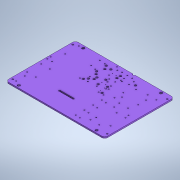
# Autodesk Inventor part: Internal Rear Plate
Saved by Autodesk Inventor 2021 (Build 250183000, 183)
## iProperties
Created: 2020-07-02
Part Number: Internal Rear Plate
Material: Generic
Document SubType Name: Modeling
Designer: jgray
Density: 1 g/cm^3
Appearance: Default
Author: jgray
Autodesk Inventor part; units mm, degrees
ref_plane "YZ Plane" through (0, 0, 0) normal (1, 0, 0) x (0, 1, 0)
ref_plane "XZ Plane" through (0, 0, 0) normal (0, 1, 0) x (-1, 0, 0)
ref_plane "XY Plane" through (0, 0, 0) normal (0, 0, 1) x (1, 0, 0)
sketch "Sketch1" plane through (0, 0, 0) normal (0, 1, 0) x (-1, 0, 0)
  line L0 (165, -123) -> (-165, -123)
  line L1 (-175, -113) -> (-175, 113)
  line L2 (-165, 123) -> (165, 123)
  line L3 (175, 113) -> (175, -113)
  line L4 (175, -123) -> (-175, 123) construction
  line L5 (-175, -123) -> (175, 123) construction
  arc A0 (165, -123) -> (175, -113) centre (165, -113) ccw
  arc A1 (175, 113) -> (165, 123) centre (165, 113) ccw
  arc A2 (-165, 123) -> (-175, 113) centre (-165, 113) ccw
  arc A3 (-175, -113) -> (-165, -123) centre (-165, -113) ccw
  line L6 (-137.85, 113.9) -> (137.85, 113.9) construction
  line L7 (137.85, 113.9) -> (137.85, -113.9) construction
  line L8 (137.85, -113.9) -> (-137.85, -113.9) construction
  line L9 (-137.85, -113.9) -> (-137.85, 113.9) construction
  line L10 (-137.85, 113.9) -> (137.85, -113.9) construction
  line L11 (137.85, 113.9) -> (-137.85, -113.9) construction
  line L12 (137.85, -114.5) -> (137.85, -113.3) construction
  line L13 (142.05, -114.5) -> (142.05, -113.3)
  line L14 (133.65, -113.3) -> (133.65, -114.5)
  arc A4 (133.65, -114.5) -> (142.05, -114.5) centre (137.85, -114.5) ccw
  arc A5 (142.05, -113.3) -> (133.65, -113.3) centre (137.85, -113.3) ccw
  line L15 (137.85, 113.75) -> (137.85, 114.95) construction
  line L16 (142.05, 113.75) -> (142.05, 114.95)
  line L17 (133.65, 114.95) -> (133.65, 113.75)
  arc A6 (133.65, 113.75) -> (142.05, 113.75) centre (137.85, 113.75) ccw
  arc A7 (142.05, 114.95) -> (133.65, 114.95) centre (137.85, 114.95) ccw
  line L18 (-137.85, 113.75) -> (-137.85, 114.95) construction
  line L19 (-133.65, 113.75) -> (-133.65, 114.95)
  line L20 (-142.05, 114.95) -> (-142.05, 113.75)
  arc A8 (-142.05, 113.75) -> (-133.65, 113.75) centre (-137.85, 113.75) ccw
  arc A9 (-133.65, 114.95) -> (-142.05, 114.95) centre (-137.85, 114.95) ccw
  line L21 (-137.85, -114.95) -> (-137.85, -113.75) construction
  line L22 (-133.65, -114.95) -> (-133.65, -113.75)
  line L23 (-142.05, -113.75) -> (-142.05, -114.95)
  arc A10 (-142.05, -114.95) -> (-133.65, -114.95) centre (-137.85, -114.95) ccw
  arc A11 (-133.65, -113.75) -> (-142.05, -113.75) centre (-137.85, -113.75) ccw
  point P0 (0, 0)
  point P1 (0, 0)
  point P2 (137.85, 114.35)
  point P3 (-137.85, 114.35)
  point P4 (-137.85, -114.35)
  dimension "d31" = 350
  dimension "d32" = 246
  dimension "d33" = 10
  dimension "d34" = 275.7
  dimension "d35" = 227.8
  dimension "d396" = 8.4
  dimension "d397" = 0.6
  dimension "d398" = 8.4
  dimension "d399" = 0.6
  dimension "d400" = 8.4
  dimension "d401" = 0.6
  dimension "d402" = 8.4
  dimension "d403" = 0.6
  dimension "d404" = 9.1
  dimension "d405" = 9.1
  constraints: 56 end point, 24 point on circle, 24 tangent, 12 centre point, 9 point on line, 8 parallel, 4 midpoint, 3 equal radius, 2 horizontal, 2 perpendicular
  measures "d31" distance of L4.start L5.start
  measures "d32" distance between parallel lines of L0 L2
  measures "d33" radius of A0
  measures "d34" distance of L7.end L8.end
  measures "d35" distance of L6.end L7.end
  measures "d396" diameter of A5
  measures "d397" distance of L12.end L7.end
  measures "d398" diameter of A7
  measures "d399" distance of L15.end point (137.85, 114.35)
  measures "d400" diameter of A9
  measures "d401" distance of L18.end point (-137.85, 114.35)
  measures "d402" diameter of A11
  measures "d403" distance of L21.end point (-137.85, -114.35)
  measures "d404" distance between parallel lines of L2 L6
  measures "d405" distance between parallel lines of L0 L8
extrude "Extrusion1" add sketch "Sketch1" along normal blind 5
sketch "Sketch2" plane through (0, 5, 0) normal (0, 1, 0) x (1, 0, 0)
  line L0 (-165, -123) -> (165, -123) projected
  arc A0 (165, -123) -> (175, -113) centre (165, -113) ccw projected
  line L1 (175, -113) -> (175, 113) projected
  arc A1 (175, 113) -> (165, 123) centre (165, 113) ccw projected
  line L2 (165, 123) -> (-165, 123) projected
  arc A2 (-165, 123) -> (-175, 113) centre (-165, 113) ccw projected
  line L3 (-175, 113) -> (-175, -113) projected
  arc A3 (-175, -113) -> (-165, -123) centre (-165, -113) ccw projected
  line L4 (167.5, -106.5) -> (-167.5, -106.5)
  line L5 (-167.5, -106.5) -> (-167.5, 106.5)
  line L6 (-167.5, 106.5) -> (167.5, 106.5)
  line L7 (167.5, 106.5) -> (167.5, -106.5)
  line L8 (167.5, -106.5) -> (-167.5, 106.5) construction
  line L9 (-167.5, -106.5) -> (167.5, 106.5) construction
  point P0 (0, 0)
  dimension "d40" = 335
  dimension "d41" = 213
  constraints: 12 end point, 4 coincident, 2 midpoint, 2 parallel, 1 horizontal, 1 perpendicular
  measures "d40" distance of L5.end L6.end
  measures "d41" distance of L4.end L5.end
hole "Hole1" at (-167.5, 5, -106.5) at (167.5, 5, -106.5) at (167.5, 5, 106.5) at (-167.5, 5, 106.5) direction (0, -1, 0) diameter 5.6 end through all
sketch "Sketch5" plane through (0, 5, 0) normal (0, 1, 0) x (1, 0, 0)
  line L0 (150.75, 85) -> (119.75, 85) construction
  line L1 (119.75, -25) -> (150.75, -25) construction
  line L2 (199.9056, 0) -> (-194.4013, 0) construction
  line L3 (175, -113) -> (175, 113) projected
  point P0 (0, 0)
  point P1 (158, 0)
  dimension "d72" = 31
  dimension "d106" = 85
  dimension "d107" = 25
  dimension "d108" = 31
  dimension "d109" = 24.25
  dimension "d110" = 24.25
  constraints: 6 end point, 4 coincident, 2 horizontal, 2 point on line
  measures "d72" distance of L1.end L1.start
  measures "d106" distance from line of point (150.75, 85) L2
  measures "d107" distance between parallel lines of L2 L1
  measures "d108" distance of L0.start L0.end
  measures "d109" distance from line of L3 point (150.75, 85)
  measures "d110" distance from line of L3 point (150.75, -25)
hole "Hole3" at (150.75, 5, -85) at (119.75, 5, -85) at (150.75, 5, 25) at (119.75, 5, 25) direction (0, -1, 0) diameter 3.8 end through all
sketch "Sketch6" plane through (0, 5, 0) normal (0, 1, 0) x (1, 0, 0)
  line L0 (195.402, -93) -> (-63.7996, -93) construction
  line L1 (204.9094, 9) -> (-63.7996, 9) construction
  line L2 (-165, -123) -> (165, -123) construction
  line L3 (165, 123) -> (-165, 123) construction
  line L4 (175, -113) -> (175, 113) construction
  point P0 (0, 0)
  point P1 (195.402, -93)
  point P2 (-63.7996, -93)
  point P3 (204.9094, 9)
  point P4 (-63.7996, 9)
  point P5 (94.75, 9)
  point P6 (94.75, -93)
  point P7 (125.75, 9)
  point P8 (125.75, -93)
  dimension "d82" = 30
  dimension "d83" = 114
  dimension "d84" = 80.25
  dimension "d85" = 80.25
  dimension "d86" = 31
  dimension "d87" = 31
  dimension "d133" = 102
  constraints: 10 other
  measures "d84" distance from line of L4 point (94.75, 9)
  measures "d85" distance from line of point (94.75, -93) L4
  measures "d86" distance of point (94.75, 9) point (125.75, 9)
  measures "d87" distance of point (94.75, -93) point (125.75, -93)
  measures "d133" distance of point (125.75, -93) point (125.75, 9)
hole "Hole4" at (94.75, 5, -9) at (94.75, 5, 93) at (125.75, 5, -9) at (125.75, 5, 93) direction (0, -1, 0) diameter 3.8 end through all
sketch "Sketch7" plane through (0, 5, 0) normal (0, 1, 0) x (1, 0, 0)
  line L0 (-55.6475, -59) -> (-200.9918, -59) construction
  line L1 (-55.6475, -9) -> (-204.5492, -9) construction
  line L2 (-133.25, -141.7869) -> (-133.25, 81.8197) construction
  line L3 (-164.25, -146.3607) -> (-164.25, 53.8689) construction
  line L4 (-175, 113) -> (-175, -113) construction
  line L5 (-165, -123) -> (165, -123) construction
  point P0 (0, 0)
  point P1 (-164.25, -9)
  point P2 (-133.25, -9)
  point P3 (-133.25, -59)
  point P4 (-164.25, -59)
  dimension "d95" = 31
  dimension "d96" = 41.75
  dimension "d97" = 64
  dimension "d98" = 50
  constraints: 8 end point, 8 point on line, 2 horizontal, 2 vertical
  measures "d95" distance between parallel lines of L3 L2
  measures "d96" distance between parallel lines of L4 L2
  measures "d97" distance between parallel lines of L5 L0
  measures "d98" distance between parallel lines of L0 L1
hole "Hole5" at (-164.25, 5, 9) at (-133.25, 5, 9) at (-133.25, 5, 59) at (-164.25, 5, 59) direction (0, -1, 0) diameter 3.8 end through all
sketch "Sketch8" plane through (0, 5, 0) normal (0, 1, 0) x (1, 0, 0)
  line L0 (-156.25, -168.1311) -> (-156.25, 234.4364) construction
  line L1 (-175, 113) -> (-175, -113) construction
  line L2 (-165, -123) -> (165, -123) construction
  point P0 (0, 0)
  point P1 (-156.25, -106)
  point P2 (-156.25, -75)
  dimension "d111" = 18.75
  dimension "d112" = 17
  dimension "d113" = 31
  constraints: 2 end point, 2 point on line, 1 vertical
  measures "d111" distance between parallel lines of L1 L0
  measures "d112" distance from line of point (-156.25, -106) L2
  measures "d113" distance of point (-156.25, -75) point (-156.25, -106)
hole "Hole6" at (-156.25, 5, 106) at (-156.25, 5, 75) direction (0, -1, 0) diameter 3.8 end through all
sketch "Sketch9" plane through (0, 5, 0) normal (0, 1, 0) x (1, 0, 0)
  line L0 (69.75, 186.0812) -> (69.75, -151.0812) construction
  circle A0 centre (-156.25, -106) radius 1.9 construction
  circle A1 centre (-156.25, -75) radius 1.9 construction
  circle A2 centre (-133.25, -59) radius 1.9 construction
  circle A3 centre (-164.25, -9) radius 1.9 construction
  circle A4 centre (-133.25, -9) radius 1.9 construction
  circle A5 centre (-164.25, -59) radius 1.9 construction
  circle A6 centre (125.75, 9) radius 1.9 construction
  circle A7 centre (94.75, 9) radius 1.9 construction
  circle A8 centre (94.75, -93) radius 1.9 construction
  circle A9 centre (125.75, -93) radius 1.9 construction
  circle A10 centre (150.75, -25) radius 1.9 construction
  circle A11 centre (150.75, 85) radius 1.9 construction
  circle A12 centre (119.75, 85) radius 1.9 construction
  circle A13 centre (119.75, -25) radius 1.9 construction
  circle A14 centre (167.5, -106.5) radius 2.8 construction
  circle A15 centre (-167.5, 106.5) radius 2.8 construction
  circle A16 centre (167.5, 106.5) radius 2.8 construction
  circle A17 centre (-167.5, -106.5) radius 2.8 construction
  line L1 (-165, -123) -> (165, -123) construction
  arc A18 (165, -123) -> (175, -113) centre (165, -113) ccw construction
  line L2 (175, -113) -> (175, 113) construction
  arc A19 (175, 113) -> (165, 123) centre (165, 113) ccw construction
  line L3 (165, 123) -> (-165, 123) construction
  arc A20 (-165, 123) -> (-175, 113) centre (-165, 113) ccw construction
  line L4 (-175, 113) -> (-175, -113) construction
  arc A21 (-175, -113) -> (-165, -123) centre (-165, -113) ccw construction
  point P0 (0, 0)
  point P1 (69.75, -106)
  point P2 (69.75, -75)
  point P3 (69.75, 17.5)
  point P4 (69.75, 48.5)
  dimension "d121" = 226
  dimension "d122" = 17
  dimension "d123" = 31
  dimension "d131" = 123.5
  dimension "d132" = 31
  constraints: 3 point on line, 2 end point, 1 midpoint, 1 vertical
  measures "d121" distance from line of A0.centre L0
  measures "d122" distance from line of point (69.75, -106) L1
  measures "d123" distance of point (69.75, -75) point (69.75, -106)
  measures "d131" distance of point (69.75, 17.5) point (69.75, -106)
  measures "d132" distance of point (69.75, 48.5) point (69.75, 17.5)
hole "Hole7" at (69.75, 5, 106) at (69.75, 5, 75) at (69.75, 5, -48.5) at (69.75, 5, -17.5) direction (0, -1, 0) diameter 3.8 end through all
sketch "Sketch10" plane through (0, 5, 0) normal (0, 1, 0) x (1, 0, 0)
  line L0 (-152.5, 188.1856) -> (-152.5, -152.5856) construction
  line L1 (-175, 113) -> (-175, -113) construction
  line L2 (-244.4549, 5.8) -> (30.8636, 5.8) construction
  line L3 (165, 123) -> (-165, 123) construction
  point P0 (0, 0)
  point P1 (-152.5, 113)
  point P2 (-152.5, 64.4)
  point P3 (-152.5, 17.8)
  dimension "d134" = 22.5
  dimension "d135" = 117.2
  dimension "d136" = 10
  dimension "d137" = 12
  dimension "d138" = 58.6
  dimension "d139" = 46.6
  constraints: 4 end point, 2 point on line, 1 horizontal, 1 midpoint, 1 vertical
  measures "d134" distance between parallel lines of L0 L1
  measures "d135" distance between parallel lines of L3 L2
  measures "d136" distance from line of L3 point (-152.5, 113)
  measures "d137" distance from line of point (-152.5, 17.8) L2
  measures "d138" distance from line of L3 point (-152.5, 64.4)
  measures "d139" distance of point (-152.5, 17.8) point (-152.5, 64.4)
hole "Hole8" at (-152.5, 5, -113) at (-152.5, 5, -64.4) at (-152.5, 5, -17.8) direction (0, -1, 0) diameter 3.8 end through all
sketch "Sketch11" plane through (0, 5, 0) normal (0, 1, 0) x (1, 0, 0)
  line L0 (-43.35, 174.5483) -> (-43.35, -176.0329) construction
  line L1 (-175, 113) -> (-175, -113) construction
  line L2 (-284.7613, 100.837) -> (238.57, 100.837) construction
  line L3 (-280.9506, 66.7) -> (255.0829, 66.7) construction
  line L4 (-280.9506, 19.8) -> (255.0829, 19.8) construction
  line L5 (-165, -123) -> (165, -123) construction
  line L6 (165, 123) -> (-165, 123) projected
  point P0 (0, 0)
  point P1 (-43.35, 19.8)
  point P2 (-43.35, 66.7)
  point P3 (-43.35, 100.837)
  dimension "d148" = 131.65
  dimension "d182" = 22.163
  dimension "d184" = 56.3
  dimension "d185" = 103.2
  constraints: 8 end point, 6 point on line, 3 horizontal, 1 vertical
  measures "d148" distance between parallel lines of L0 L1
  measures "d182" distance between parallel lines of L6 L2
  measures "d184" distance from line of point (-43.35, 66.7) L6
  measures "d185" distance from line of point (-43.35, 19.8) L6
hole "Hole9" at (-43.35, 5, -19.8) at (-43.35, 5, -66.7) at (-43.35, 5, -100.837) direction (0, -1, 0) diameter 7.5 end through all
sketch "Sketch12" plane through (0, 5, 0) normal (0, 1, 0) x (1, 0, 0)
  line L0 (-35.4, 151.1393) -> (-35.4, -165.813) construction
  line L1 (-227.4427, 87.7) -> (39.619, 87.7) construction
  line L2 (-224.5079, 56.8) -> (32.5757, 56.8) construction
  line L3 (-224.5079, 29.7) -> (32.5757, 29.7) construction
  line L4 (-175, 113) -> (-175, -113) construction
  line L5 (-165, -123) -> (165, -123) construction
  line L6 (165, 123) -> (-165, 123) projected
  point P0 (0, 0)
  point P1 (-35.4, 29.7)
  point P2 (-35.4, 56.8)
  point P3 (-35.4, 87.7)
  dimension "d159" = 139.6
  dimension "d186" = 35.3
  dimension "d187" = 66.2
  dimension "d188" = 93.3
  constraints: 8 end point, 6 point on line, 3 horizontal, 1 vertical
  measures "d159" distance between parallel lines of L0 L4
  measures "d186" distance from line of L6 point (-35.4, 87.7)
  measures "d187" distance from line of L6 point (-35.4, 56.8)
  measures "d188" distance from line of L6 point (-35.4, 29.7)
hole "Hole10" at (-35.4, 5, -29.7) at (-35.4, 5, -56.8) at (-35.4, 5, -87.7) direction (0, -1, 0) diameter 7.5 end through all
sketch "Sketch13" plane through (0, 5, 0) normal (0, 1, 0) x (1, 0, 0)
  line L0 (-23.75, 147.6176) -> (-23.75, -176.9651) construction
  line L1 (-23.75, 147.6176) -> (-23.75, -183.4215) construction
  line L2 (-211.595, 38.3) -> (40.206, 38.3) construction
  line L3 (-206.3125, 48.2) -> (33.7496, 48.2) construction
  line L4 (-189.3866, 97.6) -> (48.9146, 97.6) construction
  line L5 (-175, 113) -> (-175, -113) construction
  line L6 (-165, -123) -> (165, -123) construction
  line L7 (165, 123) -> (-165, 123) projected
  point P0 (0, 0)
  point P1 (-23.75, 38.3)
  point P2 (-23.75, 48.2)
  point P3 (-23.75, 97.6)
  dimension "d170" = 151.25
  dimension "d171" = 151.25
  dimension "d189" = 25.4
  dimension "d190" = 74.8
  dimension "d191" = 84.7
  constraints: 10 end point, 6 point on line, 3 horizontal, 2 vertical
  measures "d170" distance between parallel lines of L0 L5
  measures "d171" distance between parallel lines of L1 L5
  measures "d189" distance from line of L7 point (-23.75, 97.6)
  measures "d190" distance from line of L7 point (-23.75, 48.2)
  measures "d191" distance from line of L7 point (-23.75, 38.3)
hole "Hole11" at (-23.75, 5, -38.3) at (-23.75, 5, -48.2) at (-23.75, 5, -97.6) direction (0, -1, 0) diameter 7.5 end through all
sketch "Sketch14" plane through (0, 5, 0) normal (0, 1, 0) x (1, 0, 0)
  line L0 (-0.75, 178.7259) -> (-0.75, -161.1174) construction
  line L1 (-219.2254, 56.8) -> (83.6402, 56.8) construction
  line L2 (-209.8342, 29.7) -> (83.6402, 29.7) construction
  line L3 (-175, 113) -> (-175, -113) construction
  line L4 (165, 123) -> (-165, 123) construction
  point P0 (0, 0)
  point P1 (-0.75, 56.8)
  point P2 (-0.75, 29.7)
  dimension "d192" = 174.25
  dimension "d193" = 66.2
  dimension "d194" = 93.3
  constraints: 6 end point, 4 point on line, 2 horizontal, 1 vertical
  measures "d192" distance between parallel lines of L0 L3
  measures "d193" distance between parallel lines of L1 L4
  measures "d194" distance between parallel lines of L2 L4
hole "Hole12" at (-0.75, 5, -56.8) at (-0.75, 5, -29.7) direction (0, -1, 0) diameter 7.5 end through all
sketch "Sketch15" plane through (0, 5, 0) normal (0, 1, 0) x (1, 0, 0)
  line L0 (23.85, 172.8564) -> (23.85, -165.2261) construction
  line L1 (13.85, 166.9869) -> (13.85, -170.5086) construction
  line L2 (-225.0949, 38.3) -> (230.9643, 38.3) construction
  line L3 (-217.4645, 81.65) -> (223.334, 81.65) construction
  line L4 (-230.3774, 93.95) -> (265.0074, 93.95) construction
  line L5 (165, 123) -> (-165, 123) construction
  line L6 (-175, 113) -> (-175, -113) construction
  point P0 (0, 0)
  point P1 (23.85, 38.3)
  point P2 (13.85, 81.65)
  point P3 (13.85, 93.95)
  dimension "d202" = 29.05
  dimension "d203" = 41.35
  dimension "d204" = 84.7
  dimension "d205" = 198.85
  dimension "d206" = 188.85
  constraints: 10 end point, 6 point on line, 3 horizontal, 2 vertical
  measures "d202" distance between parallel lines of L5 L4
  measures "d203" distance between parallel lines of L3 L5
  measures "d204" distance between parallel lines of L2 L5
  measures "d205" distance between parallel lines of L0 L6
  measures "d206" distance between parallel lines of L1 L6
hole "Hole13" at (23.85, 5, -38.3) at (13.85, 5, -81.65) at (13.85, 5, -93.95) direction (0, -1, 0) diameter 7.5 end through all
sketch "Sketch16" plane through (0, 5, 0) normal (0, 1, 0) x (1, 0, 0)
  line L0 (69.203, 158.1827) -> (69.203, -196.9213) construction
  line L1 (-225.6818, 92.24) -> (239.7686, 92.24) construction
  line L2 (33.1, 158.1827) -> (33.1, -196.9213) construction
  line L3 (-211.0081, 122.771) -> (219.2254, 122.771) construction
  line L4 (-214.5298, 9.961) -> (242.7033, 9.961) construction
  line L5 (-175, 113) -> (-175, -113) construction
  line L6 (165, 123) -> (-165, 123) construction
  point P0 (0, 0)
  point P1 (69.203, 92.24)
  point P2 (33.1, 9.961)
  point P3 (33.1, 122.771)
  dimension "d214" = 244.203
  dimension "d215" = 30.76
  dimension "d216" = 0.229
  dimension "d217" = 113.039
  dimension "d218" = 208.1
  constraints: 10 end point, 6 point on line, 3 horizontal, 2 vertical
  measures "d214" distance between parallel lines of L0 L5
  measures "d215" distance between parallel lines of L6 L1
  measures "d216" distance between parallel lines of L3 L6
  measures "d217" distance between parallel lines of L4 L6
  measures "d218" distance between parallel lines of L2 L5
hole "Hole14" at (69.203, 5, -92.24) at (33.1, 5, -9.961) at (33.1, 5, -122.771) direction (0, -1, 0) diameter 7.5 end through all
sketch "Sketch17" plane through (0, 5, 0) normal (0, 1, 0) x (1, 0, 0)
  line L0 (8.45, 164.0522) -> (8.45, -151.7263) construction
  line L1 (27.7, 180.2414) -> (27.7, -141.4065) construction
  line L2 (-208.0733, 93.021) -> (246.225, 93.021) construction
  line L3 (-197.5083, 82.221) -> (249.7467, 82.221) construction
  line L4 (-203.9647, 53.6) -> (256.2031, 53.6) construction
  line L5 (29.357, 123) -> (-165, 123) construction
  line L6 (-175, 113) -> (-175, -113) construction
  point P0 (0, 0)
  point P1 (27.7, 93.021)
  point P2 (27.7, 82.221)
  point P3 (8.45, 53.6)
  dimension "d226" = 29.979
  dimension "d227" = 40.779
  dimension "d228" = 69.4
  dimension "d229" = 183.45
  dimension "d230" = 202.7
  constraints: 10 end point, 6 point on line, 3 horizontal, 2 vertical
  measures "d226" distance between parallel lines of L5 L2
  measures "d227" distance between parallel lines of L3 L5
  measures "d228" distance from line of L4.start L5
  measures "d229" distance between parallel lines of L0 L6
  measures "d230" distance between parallel lines of L1 L6
hole "Hole15" at (27.7, 5, -93.021) at (27.7, 5, -82.221) at (8.45, 5, -53.6) direction (0, -1, 0) diameter 3.8 end through all
sketch "Sketch18" plane through (0, 5, 0) normal (0, 1, 0) x (1, 0, 0)
  line L0 (22.35, 162.8783) -> (22.35, -189.291) construction
  line L1 (-211.595, 28.951) -> (225.0949, 28.951) construction
  line L2 (-219.2254, 15.483) -> (229.2035, 15.483) construction
  line L3 (-175, 113) -> (-175, -113) construction
  line L4 (29.357, 123) -> (-165, 123) construction
  point P0 (0, 0)
  point P1 (22.35, 28.951)
  point P2 (22.35, 15.483)
  dimension "d238" = 197.35
  dimension "d239" = 94.049
  dimension "d240" = 107.517
  constraints: 6 end point, 4 point on line, 2 horizontal, 1 vertical
  measures "d238" distance between parallel lines of L0 L3
  measures "d239" distance between parallel lines of L1 L4
  measures "d240" distance between parallel lines of L2 L4
hole "Hole16" at (22.35, 5, -28.951) at (22.35, 5, -15.483) direction (0, -1, 0) diameter 1.85 end through all
sketch "Sketch19" plane through (0, 5, 0) normal (0, 1, 0) x (1, 0, 0)
  line L0 (-286.1375, 42.132) -> (254.4423, 42.132) construction
  line L1 (13.471, 165.813) -> (13.471, -183.4215) construction
  line L2 (0.003, 162.2913) -> (0.003, -195.1605) construction
  line L3 (29.357, 123) -> (-165, 123) construction
  line L4 (-175, 113) -> (-175, -113) construction
  point P0 (0, 0)
  point P1 (0.003, 42.132)
  point P2 (13.471, 42.132)
  dimension "d248" = 80.868
  dimension "d249" = 175.003
  dimension "d250" = 188.471
  constraints: 6 end point, 4 point on line, 2 vertical, 1 horizontal
  measures "d248" distance between parallel lines of L0 L3
  measures "d249" distance between parallel lines of L2 L4
  measures "d250" distance between parallel lines of L1 L4
hole "Hole17" at (0.003, 5, -42.132) at (13.471, 5, -42.132) direction (0, -1, 0) diameter 1.85 end through all
sketch "Sketch20" plane through (0, 5, 0) normal (0, 1, 0) x (1, 0, 0)
  line L0 (-255.6162, 87.839) -> (262.6596, 87.839) construction
  line L1 (5.073, 175.7912) -> (5.073, -149.3785) construction
  line L2 (-8.395, 171.6825) -> (-8.395, -155.8349) construction
  line L3 (29.357, 123) -> (-165, 123) construction
  line L4 (-175, 113) -> (-175, -113) construction
  point P0 (0, 0)
  point P1 (-8.395, 87.839)
  point P2 (5.073, 87.839)
  dimension "d258" = 35.161
  dimension "d259" = 180.073
  dimension "d260" = 166.605
  constraints: 6 end point, 4 point on line, 2 vertical, 1 horizontal
  measures "d258" distance between parallel lines of L0 L3
  measures "d259" distance between parallel lines of L1 L4
  measures "d260" distance between parallel lines of L2 L4
hole "Hole18" at (-8.395, 5, -87.839) at (5.073, 5, -87.839) direction (0, -1, 0) diameter 1.85 end through all
sketch "Sketch21" plane through (0, 5, 0) normal (0, 1, 0) x (1, 0, 0)
  line L0 (-51.95, 164.0522) -> (-51.95, -151.7263) construction
  circle A0 centre (-43.35, 100.837) radius 3.75 construction
  line L1 (-62.0295, 16.1) -> (-39.6, 16.1) construction
  line L2 (-59.1779, 70.4) -> (-36.7216, 70.4) construction
  line L3 (-62.0295, 104.537) -> (-36.7216, 104.537) construction
  circle A1 centre (-43.35, 19.8) radius 3.75 construction
  circle A2 centre (-43.35, 66.7) radius 3.75 construction
  circle A3 centre (-35.4, 87.7) radius 3.75 construction
  circle A4 centre (-35.4, 29.7) radius 3.75 construction
  point P0 (0, 0)
  point P1 (-51.95, 70.4)
  point P2 (-51.95, 16.1)
  point P3 (-20.9, 116.3)
  point P4 (-39.1, 38.3)
  point P5 (-51.95, 104.537)
  dimension "d268" = 8.6
  dimension "d269" = 3.7
  dimension "d270" = 3.7
  dimension "d271" = 3.7
  dimension "d275" = 3.7
  dimension "d276" = 8.6
  dimension "d277" = 28.6
  dimension "d278" = 14.5
  constraints: 8 end point, 6 point on line, 3 horizontal, 1 vertical
  measures "d268" distance from line of A0.centre L0
  measures "d269" distance from line of L1 A1.centre
  measures "d270" distance from line of A2.centre L2
  measures "d271" distance from line of A0.centre L3
  measures "d275" horizontal distance of A4.centre point (-39.1, 38.3)
  measures "d276" vertical distance of point (-39.1, 38.3) A4.centre
  measures "d277" vertical distance of point (-20.9, 116.3) A3.centre
  measures "d278" horizontal distance of point (-20.9, 116.3) A3.centre
hole "Hole19" at (-51.95, 5, -70.4) at (-51.95, 5, -16.1) at (-20.9, 5, -116.3) at (-39.1, 5, -38.3) at (-51.95, 5, -104.537) direction (0, -1, 0) diameter 3.8 end through all
sketch "Sketch22" plane through (0, 5, 0) normal (0, 1, 0) x (1, 0, 0)
  circle A0 centre (-23.75, 97.6) radius 3.75 projected
  circle A1 centre (-23.75, 38.3) radius 3.75 projected
  point P0 (0, 0)
  point P1 (-9.25, 106.2)
  point P2 (-9.25, 76.8)
  point P3 (-27.45, 19.7)
  dimension "d286" = 14.5
  dimension "d287" = 14.5
  dimension "d288" = 8.6
  dimension "d289" = 20.8
  dimension "d290" = 18.6
  dimension "d291" = 3.7
  measures "d286" horizontal distance of A0.centre point (-9.25, 106.2)
  measures "d287" horizontal distance of A0.centre point (-9.25, 76.8)
  measures "d288" vertical distance of point (-9.25, 106.2) A0.centre
  measures "d289" vertical distance of A0.centre point (-9.25, 76.8)
  measures "d290" vertical distance of A1.centre point (-27.45, 19.7)
  measures "d291" horizontal distance of point (-27.45, 19.7) A1.centre
hole "Hole20" at (-9.25, 5, -106.2) at (-9.25, 5, -76.8) at (-27.45, 5, -19.7) direction (0, -1, 0) diameter 3.8 end through all
sketch "Sketch23" plane through (0, 5, 0) normal (0, 1, 0) x (1, 0, 0)
  circle A0 centre (-0.75, 56.8) radius 3.75 projected
  circle A1 centre (-0.75, 29.7) radius 3.75 projected
  point P0 (0, 0)
  point P1 (2.95, 65.4)
  point P2 (2.95, 21.1)
  dimension "d299" = 8.6
  dimension "d300" = 8.6
  dimension "d301" = 3.7
  dimension "d302" = 3.7
  measures "d299" vertical distance of point (2.95, 65.4) A0.centre
  measures "d300" vertical distance of point (2.95, 21.1) A1.centre
  measures "d301" horizontal distance of A1.centre point (2.95, 21.1)
  measures "d302" horizontal distance of point (2.95, 65.4) A0.centre
hole "Hole21" at (2.95, 5, -65.4) at (2.95, 5, -21.1) direction (0, -1, 0) diameter 3.8 end through all
sketch "Sketch24" plane through (0, 5, 0) normal (0, 1, 0) x (1, 0, 0)
  circle A0 centre (13.85, 93.95) radius 3.75 projected
  circle A1 centre (13.85, 81.65) radius 3.75 projected
  circle A2 centre (23.85, 38.3) radius 3.75 projected
  circle A3 centre (33.1, 9.961) radius 3.75 projected
  point P0 (0, 0)
  point P1 (5.25, 108.45)
  point P2 (22.45, 67.15)
  point P3 (27.55, 46.9)
  point P4 (27.55, 29.7)
  point P5 (24.5, 6.261)
  point P6 (41.7, 6.261)
  dimension "d310" = 14.5
  dimension "d311" = 8.6
  dimension "d312" = 14.5
  dimension "d313" = 8.6
  dimension "d314" = 8.6
  dimension "d315" = 8.6
  dimension "d316" = 3.7
  dimension "d317" = 3.7
  dimension "d318" = 3.7
  dimension "d319" = 3.7
  dimension "d320" = 8.6
  dimension "d321" = 8.6
  measures "d310" vertical distance of A0.centre point (5.25, 108.45)
  measures "d311" horizontal distance of A0.centre point (5.25, 108.45)
  measures "d312" vertical distance of A1.centre point (22.45, 67.15)
  measures "d313" horizontal distance of point (22.45, 67.15) A1.centre
  measures "d314" vertical distance of point (27.55, 46.9) A2.centre
  measures "d315" vertical distance of point (27.55, 29.7) A2.centre
  measures "d316" horizontal distance of point (27.55, 29.7) A2.centre
  measures "d317" horizontal distance of point (27.55, 46.9) A2.centre
  measures "d318" vertical distance of A3.centre point (24.5, 6.261)
  measures "d319" vertical distance of A3.centre point (41.7, 6.261)
  measures "d320" horizontal distance of point (41.7, 6.261) A3.centre
  measures "d321" horizontal distance of point (24.5, 6.261) A3.centre
hole "Hole22" at (5.25, 5, -108.45) at (22.45, 5, -67.15) at (27.55, 5, -46.9) at (27.55, 5, -29.7) at (24.5, 5, -6.261) at (41.7, 5, -6.261) direction (0, -1, 0) diameter 3.8 end through all
sketch "Sketch25" plane through (0, 5, 0) normal (0, 1, 0) x (1, 0, 0)
  arc A0 (29.357, 123) -> (36.843, 123) centre (33.1, 122.771) ccw projected
  circle A1 centre (69.203, 92.24) radius 3.75 projected
  point P0 (0, 0)
  point P1 (24.5, 108.271)
  point P2 (41.7, 108.271)
  point P3 (54.703, 100.84)
  point P4 (54.703, 83.64)
  dimension "d329" = 8.6
  dimension "d330" = 8.6
  dimension "d331" = 14.5
  dimension "d332" = 14.5
  dimension "d333" = 14.5
  dimension "d334" = 14.5
  dimension "d335" = 8.6
  dimension "d336" = 8.6
  measures "d329" horizontal distance of point (24.5, 108.271) A0.centre
  measures "d330" horizontal distance of A0.centre point (41.7, 108.271)
  measures "d331" vertical distance of A0.centre point (41.7, 108.271)
  measures "d332" vertical distance of A0.centre point (24.5, 108.271)
  measures "d333" horizontal distance of A1.centre point (54.703, 83.64)
  measures "d334" horizontal distance of A1.centre point (54.703, 100.84)
  measures "d335" vertical distance of A1.centre point (54.703, 83.64)
  measures "d336" vertical distance of A1.centre point (54.703, 100.84)
hole "Hole23" at (24.5, 5, -108.271) at (41.7, 5, -108.271) at (54.703, 5, -100.84) at (54.703, 5, -83.64) direction (0, -1, 0) diameter 3.8 end through all
sketch "Sketch26" plane through (0, 5, 0) normal (0, 1, 0) x (1, 0, 0)
  line L0 (-175, 113) -> (-175, -113) projected
  line L1 (165, 123) -> (36.843, 123) projected
  line L2 (29.357, 123) -> (-165, 123) projected
  line L3 (27.775, 30) -> (135.725, 30) construction
  line L4 (135.725, 30) -> (135.725, 83.34) construction
  line L5 (135.725, 83.34) -> (27.775, 83.34) construction
  line L6 (27.775, 83.34) -> (27.775, 30) construction
  point P0 (0, 0)
  point P1 (33.275, 80)
  point P2 (33.275, 33)
  point P3 (82.385, 80.8)
  point P4 (81.115, 32.518)
  point P5 (133.185, 65.56)
  point P6 (133.185, 37.62)
  dimension "d348" = 208.275
  dimension "d349" = 208.275
  dimension "d354" = 43
  dimension "d355" = 90
  dimension "d363" = 107.95
  dimension "d364" = 53.34
  dimension "d365" = 3
  dimension "d366" = 5.5
  dimension "d367" = 3.34
  dimension "d368" = 5.5
  dimension "d370" = 2.54
  dimension "d371" = 54.61
  dimension "d372" = 53.34
  dimension "d373" = 2.54
  dimension "d374" = 2.54
  dimension "d375" = 7.62
  dimension "d376" = 17.78
  constraints: 8 end point, 2 parallel, 1 horizontal, 1 perpendicular
  measures "d348" distance from line of L0 point (33.275, 33)
  measures "d349" distance from line of L0 point (33.275, 80)
  measures "d354" distance from line of L2 point (33.275, 80)
  measures "d355" distance from line of L2 point (33.275, 33)
  measures "d363" distance between parallel lines of L4 L6
  measures "d364" distance between parallel lines of L5 L3
  measures "d365" distance from line of point (33.275, 33) L3
  measures "d366" distance from line of point (33.275, 33) L6
  measures "d367" distance from line of point (33.275, 80) L5
  measures "d368" distance from line of L6 point (33.275, 80)
  measures "d370" distance from line of L5 point (82.385, 80.8)
  measures "d371" distance from line of point (82.385, 80.8) L6
  measures "d372" distance from line of point (81.115, 32.518) L6
  measures "d373" distance from line of point (133.185, 65.56) L4
  measures "d374" distance from line of L4 point (133.185, 37.62)
  measures "d375" distance from line of L3 point (133.185, 37.62)
  measures "d376" distance from line of L5 point (133.185, 65.56)
hole "Hole24" at (33.275, 5, -80) at (33.275, 5, -33) at (82.385, 5, -80.8) at (81.115, 5, -32.518) at (133.185, 5, -65.56) at (133.185, 5, -37.62) direction (0, -1, 0) diameter 3.8 end through all
sketch "Sketch27" plane through (0, 5, 0) normal (0, 1, 0) x (1, 0, 0)
  line L0 (94, 3) -> (153, 3) construction
  line L1 (153, 3) -> (153, -88.5) construction
  line L2 (153, -88.5) -> (94, -88.5) construction
  line L3 (94, -88.5) -> (94, 3) construction
  line L4 (-175, 113) -> (-175, -113) construction
  line L5 (165, 123) -> (36.843, 123) construction
  point P0 (0, 0)
  point P1 (98, -12)
  point P2 (149, -12)
  point P3 (98, -76)
  point P4 (149, -76)
  dimension "d377" = 59
  dimension "d378" = 91.5
  dimension "d379" = 15
  dimension "d380" = 15
  dimension "d381" = 12.5
  dimension "d382" = 12.5
  dimension "d383" = 4
  dimension "d384" = 4
  dimension "d385" = 4
  dimension "d386" = 4
  dimension "d387" = 273
  dimension "d388" = 135
  constraints: 8 end point, 2 parallel, 1 horizontal, 1 perpendicular
  measures "d377" distance of L1.end L2.end
  measures "d378" distance of L0.end L1.end
  measures "d379" distance from line of point (98, -12) L0
  measures "d380" distance from line of point (149, -12) L0
  measures "d381" distance from line of L2 point (149, -76)
  measures "d382" distance from line of L2 point (98, -76)
  measures "d383" distance from line of L3 point (98, -76)
  measures "d384" distance from line of L3 point (98, -12)
  measures "d385" distance from line of L1 point (149, -12)
  measures "d386" distance from line of L1 point (149, -76)
  measures "d387" distance from line of L4 point (98, -12)
  measures "d388" distance from line of L5 point (98, -12)
hole "Hole25" at (98, 5, 12) at (149, 5, 12) at (98, 5, 76) at (149, 5, 76) direction (0, -1, 0) diameter 3.8 end through all
sketch "Sketch28" plane through (0, 5, 0) normal (0, 1, 0) x (1, 0, 0)
  line L0 (-115.5, 133.7446) -> (-115.5, -39.6343) construction
  line L1 (-175, 113) -> (-175, -113) construction
  line L2 (29.357, 123) -> (-165, 123) construction
  point P0 (0, 0)
  point P1 (-115.5, 61.75)
  dimension "d406" = 59.5
  dimension "d407" = 61.25
  constraints: 2 end point, 1 point on line, 1 vertical
  measures "d406" distance between parallel lines of L0 L1
  measures "d407" distance from line of point (-115.5, 61.75) L2
sketch "Sketch29" plane through (0, 5, 0) normal (0, 1, 0) x (1, 0, 0)
  circle A0 centre (98, -76) radius 1.9 projected
  circle A1 centre (98, -12) radius 1.9 projected
  circle A2 centre (149, -12) radius 1.9 projected
  circle A3 centre (149, -76) radius 1.9 projected
  circle A4 centre (133.185, 65.56) radius 1.9 projected
  circle A5 centre (82.385, 80.8) radius 1.9 projected
  circle A6 centre (33.275, 80) radius 1.9 projected
  circle A7 centre (33.275, 33) radius 1.9 projected
  circle A8 centre (81.115, 32.518) radius 1.9 projected
  circle A9 centre (133.185, 37.62) radius 1.9 projected
  circle A10 centre (54.703, 100.84) radius 1.9 projected
  circle A11 centre (24.5, 108.271) radius 1.9 projected
  circle A12 centre (41.7, 108.271) radius 1.9 projected
  circle A13 centre (54.703, 83.64) radius 1.9 projected
  circle A14 centre (24.5, 6.261) radius 1.9 projected
  circle A15 centre (27.55, 46.9) radius 1.9 projected
  circle A16 centre (5.25, 108.45) radius 1.9 projected
  circle A17 centre (22.45, 67.15) radius 1.9 projected
  circle A18 centre (27.55, 29.7) radius 1.9 projected
  circle A19 centre (41.7, 6.261) radius 1.9 projected
  circle A20 centre (2.95, 65.4) radius 1.9 projected
  circle A21 centre (2.95, 21.1) radius 1.9 projected
  circle A22 centre (-9.25, 76.8) radius 1.9 projected
  circle A23 centre (-9.25, 106.2) radius 1.9 projected
  circle A24 centre (-27.45, 19.7) radius 1.9 projected
  circle A25 centre (-39.1, 38.3) radius 1.9 projected
  circle A26 centre (-51.95, 16.1) radius 1.9 projected
  circle A27 centre (-51.95, 70.4) radius 1.9 projected
  circle A28 centre (-20.9, 116.3) radius 1.9 projected
  circle A29 centre (-51.95, 104.537) radius 1.9 projected
  circle A30 centre (-8.395, 87.839) radius 0.925 projected
  circle A31 centre (5.073, 87.839) radius 0.925 projected
  circle A32 centre (0.003, 42.132) radius 0.925 projected
  circle A33 centre (13.471, 42.132) radius 0.925 projected
  circle A34 centre (22.35, 28.951) radius 0.925 projected
  circle A35 centre (22.35, 15.483) radius 0.925 projected
  circle A36 centre (27.7, 82.221) radius 1.9 projected
  circle A37 centre (27.7, 93.021) radius 1.9 projected
  circle A38 centre (8.45, 53.6) radius 1.9 projected
  arc A39 (29.357, 123) -> (36.843, 123) centre (33.1, 122.771) ccw projected
  line L0 (29.357, 123) -> (-165, 123) projected
  arc A40 (-165, 123) -> (-175, 113) centre (-165, 113) ccw projected
  line L1 (-175, 113) -> (-175, -113) projected
  arc A41 (-175, -113) -> (-165, -123) centre (-165, -113) ccw projected
  line L2 (-165, -123) -> (165, -123) projected
  arc A42 (165, -123) -> (175, -113) centre (165, -113) ccw projected
  line L3 (175, -113) -> (175, 113) projected
  arc A43 (175, 113) -> (165, 123) centre (165, 113) ccw projected
  line L4 (165, 123) -> (36.843, 123) projected
  circle A44 centre (33.1, 9.961) radius 3.75 projected
  circle A45 centre (69.203, 92.24) radius 3.75 projected
  circle A46 centre (13.85, 81.65) radius 3.75 projected
  circle A47 centre (23.85, 38.3) radius 3.75 projected
  circle A48 centre (13.85, 93.95) radius 3.75 projected
  circle A49 centre (-0.75, 56.8) radius 3.75 projected
  circle A50 centre (-0.75, 29.7) radius 3.75 projected
  circle A51 centre (-23.75, 48.2) radius 3.75 projected
  circle A52 centre (-23.75, 38.3) radius 3.75 projected
  circle A53 centre (-23.75, 97.6) radius 3.75 projected
  circle A54 centre (-35.4, 56.8) radius 3.75 projected
  circle A55 centre (-35.4, 29.7) radius 3.75 projected
  circle A56 centre (-35.4, 87.7) radius 3.75 projected
  circle A57 centre (-43.35, 66.7) radius 3.75 projected
  circle A58 centre (-43.35, 19.8) radius 3.75 projected
  circle A59 centre (-43.35, 100.837) radius 3.75 projected
  circle A60 centre (-152.5, 64.4) radius 1.9 projected
  circle A61 centre (-152.5, 113) radius 1.9 projected
  circle A62 centre (-152.5, 17.8) radius 1.9 projected
  circle A63 centre (69.75, 48.5) radius 1.9 projected
  circle A64 centre (69.75, -106) radius 1.9 projected
  circle A65 centre (69.75, -75) radius 1.9 projected
  circle A66 centre (69.75, 17.5) radius 1.9 projected
  circle A67 centre (-156.25, -106) radius 1.9 projected
  circle A68 centre (-156.25, -75) radius 1.9 projected
  circle A69 centre (-133.25, -59) radius 1.9 projected
  circle A70 centre (-164.25, -9) radius 1.9 projected
  circle A71 centre (-133.25, -9) radius 1.9 projected
  circle A72 centre (-164.25, -59) radius 1.9 projected
  circle A73 centre (125.75, 9) radius 1.9 projected
  circle A74 centre (94.75, 9) radius 1.9 projected
  circle A75 centre (94.75, -93) radius 1.9 projected
  circle A76 centre (125.75, -93) radius 1.9 projected
  circle A77 centre (150.75, -25) radius 1.9 projected
  circle A78 centre (150.75, 85) radius 1.9 projected
  circle A79 centre (119.75, 85) radius 1.9 projected
  circle A80 centre (119.75, -25) radius 1.9 projected
  circle A81 centre (167.5, -106.5) radius 2.8 projected
  circle A82 centre (-167.5, 106.5) radius 2.8 projected
  circle A83 centre (167.5, 106.5) radius 2.8 projected
  circle A84 centre (-167.5, -106.5) radius 2.8 projected
  arc A85 (133.65, 113.75) -> (142.05, 113.75) centre (137.85, 113.75) ccw projected
  line L5 (133.65, 113.75) -> (133.65, 114.95) projected
  arc A86 (142.05, 114.95) -> (133.65, 114.95) centre (137.85, 114.95) ccw projected
  line L6 (142.05, 114.95) -> (142.05, 113.75) projected
  arc A87 (133.65, -114.95) -> (142.05, -114.95) centre (137.85, -114.95) ccw projected
  line L7 (133.65, -114.95) -> (133.65, -113.75) projected
  arc A88 (142.05, -113.75) -> (133.65, -113.75) centre (137.85, -113.75) ccw projected
  line L8 (142.05, -113.75) -> (142.05, -114.95) projected
  arc A89 (-142.05, -114.95) -> (-133.65, -114.95) centre (-137.85, -114.95) ccw projected
  line L9 (-142.05, -114.95) -> (-142.05, -113.75) projected
  arc A90 (-133.65, -113.75) -> (-142.05, -113.75) centre (-137.85, -113.75) ccw projected
  line L10 (-133.65, -113.75) -> (-133.65, -114.95) projected
  arc A91 (-133.65, 114.5) -> (-142.05, 114.5) centre (-137.85, 114.5) ccw projected
  line L11 (-133.65, 114.5) -> (-133.65, 113.3) projected
  arc A92 (-142.05, 113.3) -> (-133.65, 113.3) centre (-137.85, 113.3) ccw projected
  line L12 (-142.05, 113.3) -> (-142.05, 114.5) projected
  line L13 (69.75, 60.55) -> (69.75, -119.15) construction
  point P0 (0, 0)
  point P1 (69.75, -44.25)
  point P2 (69.75, -13.25)
  dimension "d415" = 61.75
  dimension "d416" = 61.75
  constraints: 3 point on line, 2 end point, 1 perpendicular
  measures "d415" distance of point (69.75, -13.25) A65.centre
  measures "d416" distance of A64.centre point (69.75, -44.25)
hole "Hole27" at (69.75, 5, 44.25) at (69.75, 5, 13.25) direction (0, -1, 0) diameter 3.8 end through all
sketch "Sketch30" plane through (0, 5, 0) normal (0, 1, 0) x (1, 0, 0)
  line L0 (-186.0281, -58.75) -> (18.0462, -58.75) construction
  line L1 (-165, -123) -> (165, -123) construction
  line L2 (-50, -58.75) -> (0, -58.75) construction
  line L3 (-50, -61.275) -> (0, -61.275)
  line L4 (0, -56.225) -> (-50, -56.225)
  arc A0 (-50, -56.225) -> (-50, -61.275) centre (-50, -58.75) ccw
  arc A1 (0, -61.275) -> (0, -56.225) centre (0, -58.75) ccw
  line L5 (-50, -58.75) -> (0, -58.75) construction
  line L6 (-175, 113) -> (-175, -113) projected
  point P0 (0, 0)
  point P1 (-25, -58.75)
  dimension "d424" = 64.25
  dimension "d427" = 50
  dimension "d429" = 5.05
  dimension "d430" = 125
  constraints: 12 end point, 4 point on circle, 4 tangent, 2 centre point, 2 collinear, 2 horizontal, 1 midpoint, 1 parallel, 1 point on line
  measures "d424" distance between parallel lines of L1 L0
  measures "d427" distance of L2.start L2.end
  measures "d429" diameter of A1
  measures "d430" distance from line of L6 L2.start
extrude "Extrusion3" cut sketch "Sketch30" against normal blind 10
sketch "Sketch31" plane through (0, 5, 0) normal (0, 1, 0) x (1, 0, 0)
  line L0 (-210.3146, 5.5) -> (-120.9267, 5.5) construction
  line L1 (29.357, 123) -> (-165, 123) construction
  line L2 (-169, 134.0819) -> (-169, -28.8403) construction
  line L3 (-175, 113) -> (-175, -113) construction
  point P0 (0, 0)
  point P1 (-169, 17.5)
  point P2 (-169, 29.5)
  dimension "d433" = 117.5
  dimension "d434" = 6
  dimension "d435" = 12
  dimension "d436" = 12
  constraints: 4 end point, 2 point on line, 1 horizontal, 1 vertical
  measures "d433" distance between parallel lines of L1 L0
  measures "d434" distance between parallel lines of L3 L2
  measures "d435" distance of point (-169, 29.5) point (-169, 17.5)
  measures "d436" distance from line of L0 point (-169, 17.5)
hole "Hole28" at (-169, 5, -17.5) at (-169, 5, -29.5) direction (0, -1, 0) diameter 3.8 end through all
sketch "Sketch32" plane through (0, 5, 0) normal (0, 1, 0) x (1, 0, 0)
  line L0 (54.5, -136.4431) -> (54.5, 133.7446) construction
  line L1 (29.357, 123) -> (-165, 123) construction
  line L2 (-175, 113) -> (-175, -113) construction
  line L3 (-165, -123) -> (165, -123) projected
  line L4 (175, -113) -> (175, 113) projected
  point P0 (0, 0)
  point P1 (54.5, -105)
  point P2 (54.5, -74.25)
  point P3 (54.5, -43.25)
  point P4 (54.5, -12.5)
  dimension "d445" = 18
  dimension "d446" = 48.75
  dimension "d447" = 79.75
  dimension "d448" = 110.5
  dimension "d456" = 120.5
  constraints: 4 point on line, 2 end point, 1 perpendicular
  measures "d445" distance from line of point (54.5, -105) L3
  measures "d446" distance from line of point (54.5, -74.25) L3
  measures "d447" distance from line of L3 point (54.5, -43.25)
  measures "d448" distance from line of L3 point (54.5, -12.5)
  measures "d456" distance from line of L4 L0.start
hole "Hole29" at (54.5, 5, 105) at (54.5, 5, 74.25) at (54.5, 5, 43.25) at (54.5, 5, 12.5) direction (0, -1, 0) diameter 3.8 end through all
sketch "Sketch33" plane through (0, 5, 0) normal (0, 1, 0) x (1, 0, 0)
  line L0 (-71, 131.3834) -> (-71, 36.5984) construction
  line L1 (-175, 113) -> (-175, -113) construction
  line L2 (29.357, 123) -> (-165, 123) construction
  point P0 (0, 0)
  point P1 (-71, 106)
  point P2 (-71, 75)
  dimension "d457" = 104
  dimension "d458" = 17
  dimension "d459" = 31
  constraints: 2 end point, 2 point on line, 1 vertical
  measures "d457" distance between parallel lines of L0 L1
  measures "d458" distance from line of L2 point (-71, 106)
  measures "d459" distance of point (-71, 106) point (-71, 75)
hole "Hole30" at (-71, 5, -106) at (-71, 5, -75) direction (0, -1, 0) diameter 3.8 end through all
equation "\"d416\" = d415"
body "Solid1"
